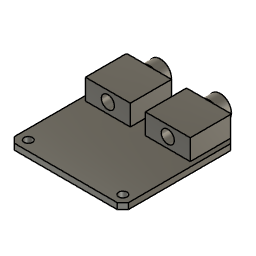
Assembly v21 (Autodesk Fusion 360 archive; units mm, degrees)
design "TEA5767"
Autodesk Fusion 360 part; units mm, degrees
sketch "Sketch1" plane through (0, 0, 0) normal (0, 0, 1) x (1, 0, 0)
  line L0 (-15.25, 15.125) -> (15.25, 15.125)
  line L1 (15.25, 15.125) -> (15.25, -15.125)
  line L2 (15.25, -15.125) -> (-15.25, -15.125)
  line L3 (-15.25, -15.125) -> (-15.25, 15.125)
  line L4 (-15.25, 15.125) -> (15.25, -15.125) construction
  line L5 (15.25, 15.125) -> (-15.25, -15.125) construction
  dimension "d1" = 30.5
  dimension "d2" = 30.25
  constraint horizontal L0
  constraint perpendicular L0 L1
  constraint parallel L0 L2
  constraint parallel L1 L3
  constraint coincident L4 origin
  constraint coincident L5 origin
  measures "d1" distance of L1.end L2.end
  measures "d2" distance of L0.end L1.end
extrude "Extrude1" add sketch "Sketch1" along normal blind 1.6
sketch "Sketch2" plane through (0, 0, 1.6) normal (0, 0, 1) x (-1, 0, 0)
  line L0 (15.25, 15.125) -> (-15.25, 15.125)
  line L1 (-15.25, 15.125) -> (-15.25, -15.125)
  line L2 (-15.25, -15.125) -> (15.25, -15.125)
  line L3 (15.25, -15.125) -> (15.25, 15.125)
  line L4 (14, -15.125) -> (2, -15.125)
  line L5 (2, -15.125) -> (2, -4.125)
  line L6 (2, -4.125) -> (14, -4.125)
  line L7 (14, -4.125) -> (14, -15.125)
  line L8 (-2, -15.125) -> (-14, -15.125)
  line L9 (-14, -15.125) -> (-14, -4.125)
  line L10 (-14, -4.125) -> (-2, -4.125)
  line L11 (-2, -4.125) -> (-2, -15.125)
  dimension "d5" = 12
  dimension "d6" = 11
  dimension "d7" = 12
  dimension "d8" = 11
  dimension "d9" = 4
  dimension "d10" = 1.25
  constraint horizontal L4
  constraint vertical L5
  constraint horizontal L6
  constraint vertical L7
  constraint coincident L2 L4.start
  constraint horizontal L8
  constraint vertical L9
  constraint horizontal L10
  constraint vertical L11
  constraint coincident L2 L8.start
  measures "d5" distance of L4.start L4.end
  measures "d6" distance of L4.start L6.end
  measures "d7" distance of L8.start L8.end
  measures "d8" distance of L8.start L10.end
  measures "d9" distance of L5 L11
  measures "d10" distance of L1 L9
extrude "Extrude2" add sketch "Sketch2" along normal blind 5.5 contours L2 L4 L5 L6 L7 | L2 L8 L9 L10 L11
sketch "Sketch3" plane through (0, 15.125, 0) normal (0, 1, 0) x (-1, 0, 0)
  line L0 (-15.25, 0) -> (15.25, 0)
  line L1 (15.25, 0) -> (15.25, 1.6)
  line L2 (15.25, 1.6) -> (14, 1.6)
  line L3 (14, 1.6) -> (14, 7.1)
  line L4 (14, 7.1) -> (2, 7.1)
  line L5 (2, 7.1) -> (2, 1.6)
  line L6 (2, 1.6) -> (-2, 1.6)
  line L7 (-2, 1.6) -> (-2, 7.1)
  line L8 (-2, 7.1) -> (-14, 7.1)
  line L9 (-14, 7.1) -> (-14, 1.6)
  line L10 (-14, 1.6) -> (-15.25, 1.6)
  line L11 (-15.25, 1.6) -> (-15.25, 0)
  line L12 (-2, 1.6) -> (-14, 7.1) construction
  line L13 (2, 1.6) -> (14, 7.1) construction
  circle A0 centre (-8, 4.35) radius 3
  circle A1 centre (8, 4.35) radius 3
  circle A2 centre (-8, 4.35) radius 1.75
  circle A3 centre (8, 4.35) radius 1.75
  dimension "d13" = 6
  dimension "d14" = 6
  dimension "d15" = 3.5
  dimension "d16" = 3.5
  constraint coincident L6.end L7.start
  constraint coincident L8.end L9.start
  constraint coincident L5.end L6.start
  constraint coincident L3.end L4.start
  constraint midpoint L12 A0.centre
  constraint midpoint L13 A1.centre
  constraint concentric A0 A2
  constraint concentric A1 A3
  measures "d13" diameter of A0
  measures "d14" diameter of A1
  measures "d15" diameter of A2
  measures "d16" diameter of A3
extrude "Extrude3" add sketch "Sketch3" along normal blind 3 contours L8 A0 | L8 A0 | L4 A1 | L4 A1
chamfer "Chamfer1" distance 1.5 angle 45 4 edges at (-15.25, -15.125, 0.8) (-15.25, 15.125, 0.8) (15.25, -15.125, 0.8) (15.25, 15.125, 0.8)
sketch "Sketch4" plane through (0, 0, 0) normal (0, 0, -1) x (1, 0, 0)
  line L0 (13.75, -15.125) -> (15.25, -13.625)
  line L1 (15.25, -13.625) -> (15.25, 13.625)
  line L2 (15.25, 13.625) -> (13.75, 15.125)
  line L3 (13.75, 15.125) -> (-13.75, 15.125)
  line L4 (-13.75, 15.125) -> (-15.25, 13.625)
  line L5 (-15.25, 13.625) -> (-15.25, -13.625)
  line L6 (-15.25, -13.625) -> (-13.75, -15.125)
  line L7 (-13.75, -15.125) -> (13.75, -15.125)
  line L8 (0, -15.125) -> (0, 15.125) construction
  circle A0 centre (0, -12.25) radius 1.125
  circle A1 centre (12.625, 12.5) radius 1.125
  circle A2 centre (-12.625, 12.5) radius 1.125
  dimension "d20" = 2.25
  dimension "d21" = 1.75
  dimension "d22" = 1.5
  dimension "d23" = 1.5
  dimension "d24" = 1.5
  dimension "d25" = 1.5
  dimension "d26" = 2.25
  dimension "d27" = 2.25
  constraint midpoint L7 L8.start
  constraint midpoint L3 L8.end
  constraint coincident L8 A0.centre
  measures "d20" diameter of A0
  measures "d21" distance of L7 A0
  measures "d22" distance of L5 A2
  measures "d23" distance of L3 A2
  measures "d24" distance of L3 A1
  measures "d25" distance of L1 A1
  measures "d26" diameter of A1
  measures "d27" diameter of A2
extrude "Extrude4" cut sketch "Sketch4" against normal blind 1.6 contours A0 | A1 | A2
extrude "Extrude5" cut 2 faces at (7.9535, 15.125, 3.807) (-7.7869, 15.125, 4.893) along direction (0, -1, 0) blind 11
equation "d10 = ( 2.5 / 2 ) * 1 mm"
